Autodesk Inventor part; units mm, degrees
(part 3 of 3)
  line L141 (-1.5109, 1.3467) -> (-1.8366, 0.452)
  arc A207 (-2.0617, 0.2877) -> (-1.8366, 0.452) centre (-2.0715, 0.5375) ccw
  arc A208 (-2.0617, 0.2877) -> (-2.0518, 0.2875) centre (-2.0518, 0.5375) ccw
  line L142 (-2.0518, 0.2875) -> (-2.0715, 0.2875)
  arc A209 (-2.0715, 0.2875) -> (-2.0617, 0.2877) centre (-2.0715, 0.5375) ccw
  arc A210 (-2.2868, 0.452) -> (-2.0617, 0.2877) centre (-2.0518, 0.5375) ccw
  line L143 (-2.2868, 0.452) -> (-2.4065, 0.7809)
  arc A211 (-2.4065, 0.7809) -> (-2.5944, 0.9125) centre (-2.5944, 0.7125) ccw
  line L144 (-2.5944, 0.9125) -> (-5.4544, 0.9125)
  line L145 (-5.4544, 0.9125) -> (-5.4544, -6.5875)
  line L146 (-5.4544, -6.5875) -> (62.5235, -6.5875)
  line L147 (62.5235, 5.2125) -> (62.5235, -6.5875)
  line L148 (50.5235, -3.6875) -> (-2.4544, -3.6875)
  arc A212 (-2.4544, -0.9875) -> (-2.4544, -3.6875) centre (-2.4544, -2.3375) ccw
  line L149 (-2.4544, -0.9875) -> (50.5235, -0.9875)
  arc A213 (50.5235, -3.6875) -> (50.5235, -0.9875) centre (50.5235, -2.3375) ccw
  line L150 (53.5235, 0.9125) -> (53.5235, -6.5875)
  point P0 (0, 0)
  constraints: 2 end point, 1 perpendicular, 1 point on line
extrude "Extrusion7" add sketch "Sketch6" along normal blind 0.2 contours L147 L146 L150 L1 L0
sketch "Sketch7" plane through (0, 0, 5.2) normal (0, 0, 1) x (1, 0, 0)
  line L0 (62.5235, 5.2125) -> (54.2115, 5.2125)
  line L1 (54.2115, 5.2125) -> (53.5235, 0.9125)
  line L2 (53.5235, 0.9125) -> (53.5235, -6.5875)
  line L3 (53.5235, -6.5875) -> (62.5235, -6.5875)
  line L4 (62.5235, -6.5875) -> (62.5235, 5.2125)
  line L5 (54.2115, 5.2125) -> (56.0035, 16.4125)
  line L6 (56.0035, 16.4125) -> (62.5235, 16.4125)
  line L7 (62.5235, 11.2125) -> (55.5235, 11.2125)
  line L8 (62.5235, 16.4125) -> (62.5235, 5.2125)
  line L9 (55.5235, 13.4125) -> (62.5235, 13.4125)
  line L10 (55.5235, 13.4125) -> (62.5235, 13.4125)
  point P0 (0, 0)
  point P1 (55.5235, 13.4125)
  dimension "d65" = 3
  constraints: 8 end point, 3 collinear, 1 parallel
  measures "d65" distance between parallel lines of L6 L9
extrude "Extrusion8" add sketch "Sketch7" along normal blind 3
sketch "Sketch10" plane through (0, 0, 5.2) normal (0, 0, -1) x (-1, 0, 0)
  line L0 (-55.5235, 13.4125) -> (-62.5235, 13.4125)
  line L1 (-62.5235, 16.4125) -> (-56.0035, 16.4125)
  line L2 (-62.5235, 16.4125) -> (-55.5235, 16.4125)
  line L3 (-55.5235, 16.4125) -> (-55.5235, 13.4125)
  line L4 (-55.5235, 13.4125) -> (-62.5235, 13.4125)
  line L5 (-62.5235, 13.4125) -> (-62.5235, 16.4125)
  point P0 (0, 0)
  constraints: 8 end point, 2 parallel, 1 horizontal, 1 perpendicular
extrude "Extrusion9" add sketch "Sketch10" along normal up to surface (5.4 mm away)
sketch "Sketch11" plane through (0, 0, 5.2) normal (0, 0, 1) x (1, 0, 0)
  line L0 (55.5235, 16.4125) -> (56.0035, 16.4125)
  line L1 (55.5235, 13.4125) -> (62.5235, 13.4125)
  line L2 (55.5235, 16.4125) -> (55.5235, 13.4125)
  line L3 (55.5235, 13.4125) -> (56.0035, 16.4125)
  line L4 (56.0035, 16.4125) -> (55.5235, 16.4125)
  point P0 (0, 0)
  constraints: 6 end point, 1 perpendicular
extrude "Extrusion10" cut sketch "Sketch11" against normal up to surface (5.4 mm away)
sketch "Sketch12" plane through (62.5235, 16.4125, -0.2) normal (0, 0, -1) x (-1, 0, 0)
  line L0 (0, 0) -> (6.52, 0)
  line L1 (8.312, -11.2) -> (7, -3.0001)
  line L2 (6.52, 0) -> (7, -3.0001)
  line L3 (7, -3) -> (0, -3)
  line L4 (7, -0.5001) -> (0, -0.5)
  line L5 (0, -3) -> (0, 0)
  point P0 (62.5235, -16.4125)
  point P1 (0, -3)
  constraints: 8 end point, 1 collinear, 1 perpendicular
extrude "Extrusion11" add sketch "Sketch12" along normal blind 10
chamfer "Chamfer3" distance 24.8 distance2 3 1 edges at (59.0235, 13.4125, -10.2) measured on face at (59.0235, 13.4125, -10.7)
sketch "Sketch13" plane through (54.2115, 5.2125, -0.2) normal (0, 1, 0) x (1, 0, 0)
  line L0 (8.312, 0) -> (0, 0)
  line L1 (8.312, 0) -> (8.312, -5.4)
  line L2 (0, 0) -> (8.312, 0)
  line L3 (8.312, 0) -> (8.312, -5.4)
  line L4 (8.312, -5.4) -> (0, -5.4)
  line L5 (0, -5.4) -> (0, 0)
  line L6 (0, 0) -> (-0.5, 0)
  line L7 (-0.5, 0) -> (-0.5, -5.4)
  line L8 (-0.5, -5.4) -> (0, -5.4)
  line L9 (0, -5.4) -> (0, 0)
  point P0 (-54.2115, -0.2)
  dimension "d92" = 0.5
  constraints: 16 end point, 4 parallel, 2 horizontal, 2 perpendicular
  measures "d92" distance of L8.end L7.end
extrude "Extrusion12" cut sketch "Sketch13" against normal blind 0.25
sketch "Sketch14" plane through (0, 0, 5) normal (0, 0, 1) x (1, 0, 0)
  line L0 (53.5235, -6.5875) -> (53.5235, 0.9125)
  line L1 (53.5235, -0.9875) -> (-5.4544, -0.9875)
  line L2 (-5.4544, -0.9875) -> (-5.4544, 1.6125)
  line L3 (-5.4544, 1.6125) -> (53.5235, 1.6125)
  line L4 (53.5235, 1.6125) -> (53.5235, -0.9875)
  line L5 (-1.1356, 1.4125) -> (-1.417, 1.4125)
  line L6 (-2.4544, -0.9875) -> (50.5235, -0.9875)
  point P0 (0, 0)
  point P1 (-1.2763, 1.4125)
  point P2 (53.5235, 0.9125)
  dimension "d79" = 0.2
  dimension "d80" = 0
  constraints: 8 end point, 2 parallel, 1 horizontal, 1 midpoint, 1 perpendicular, 1 point on line
  measures "d79" distance from line of point (-1.276, 1.413) L3
  measures "d80" distance between parallel lines of L6 L1
extrude "Extrusion13" add sketch "Sketch14" against normal blind 1
sketch "Sketch15" plane through (0, 0, 0) normal (0, 0, -1) x (-1, 0, 0)
  line L0 (-23.0711, 3.4384) -> (-23.0711, 0.0831)
  line L1 (-23.9972, 1.4125) -> (-23.7158, 1.4125)
  line L2 (-22.4264, 1.4125) -> (-22.145, 1.4125)
  point P0 (0, 0)
  point P1 (-23.8565, 1.4125)
  point P2 (-22.2857, 1.4125)
  dimension "d83" = 0.7854
  dimension "d84" = 0.7854
  constraints: 2 end point, 2 midpoint, 1 vertical
  measures "d83" distance from line of point (-23.856, 1.413) L0
  measures "d84" distance from line of point (-22.286, 1.413) L0
ref_plane "Work Plane1" through (23.0711, 3.4384, 0) normal (1, 0, 0) x (0, -1, 0)
sketch "Sketch16" plane through (-5.4544, -6.5875, 0) normal (0, -1, 0) x (1, 0, 0)
  line L0 (0, 0) -> (58.9779, 0)
  line L1 (60.9779, -14) -> (58.9779, 0)
  line L2 (60.9779, -14) -> (60.9779, -35)
  line L3 (60.9779, -35) -> (67.9779, -35)
  line L4 (67.9779, -35) -> (67.9779, 8.2)
  line L5 (58.9779, 8.2) -> (67.9779, 8.2)
  line L6 (58.9779, 5) -> (58.9779, 8.2)
  line L7 (0, 5) -> (58.9779, 5)
  line L8 (0, 0) -> (0, 5)
  line L9 (60.435, -10.2) -> (67.9779, -10.2)
  line L10 (58.9779, 5) -> (58.9779, 0)
  point P0 (5.4544, 0)
  dimension "d86" = 18.4
  constraints: 4 end point, 2 point on line, 1 perpendicular
  measures "d86" distance between parallel lines of L5 L9
extrude "Extrusion14" add sketch "Sketch16" along normal blind 3 contours L10 L6 L5 L4 L9 L1
chamfer "Chamfer4" distance 24.8 distance2 3 1 edges at (58.7521, -6.5875, -10.2) measured on face at (58.7521, -6.5875, -10.7)
sketch "Sketch17" plane through (62.5235, -6.5875, 0) normal (1, 0, 0) x (0, 0, -1)
  line L0 (10.2, 23) -> (-8.2, 23)
  line L1 (-8.2, 23) -> (-8.2, -3)
  line L2 (10.2, -3) -> (-8.2, -3)
  line L3 (35, 0) -> (10.2, -3)
  line L4 (35, 0) -> (35, 20)
  line L5 (10.2, 23) -> (35, 20)
  circle A0 centre (20, 5) radius 2.8
  circle A1 centre (30, 5) radius 2.8
  circle A2 centre (20, 15) radius 2.8
  circle A3 centre (30, 15) radius 2.8
  line L6 (0.2, 20) -> (0.2, 11.55)
  line L7 (0.2, 11.55) -> (-5.2, 11.55)
  line L8 (-5.2, 11.55) -> (-5.2, 20)
  line L9 (-5.2, 20) -> (0.2, 20)
  point P0 (0, 6.5875)
extrude "Extrusion15" add sketch "Sketch17" along normal blind 1.1
sketch "Sketch18" plane through (55.5235, 13.4124, 5.2) normal (0, -1, 0) x (1, 0, 0)
  line L0 (0, 0) -> (0, -5.4)
  line L1 (0, -5.4) -> (8.1, -5.4)
  line L2 (8.1, 0) -> (8.1, -5.4)
  line L3 (0, 0) -> (8.1, 0)
  point P0 (-55.5235, -5.2)
extrude "Extrusion16" cut sketch "Sketch18" against normal blind 0.3
equation "\"d1\" = 1.5708 * pitch"
equation "\"d2\" = 1.5708 * pitch"
equation "\"d4\" = 2.25 * pitch"
equation "\"d5\" = pitch"
equation "\"d11\" = d3"
equation "\"a_pres\" = 20deg"
equation "\"pitch\" = 0.5"
body "Solid1"
